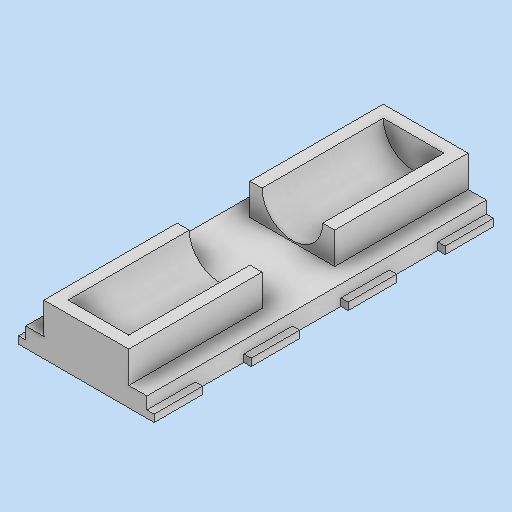
# Autodesk Inventor part: bottom plate
Saved by Autodesk Inventor 2026 (Build 300175000, 175)
## iProperties
Created: 2026-02-10
Part Number: bottom plate
Material: Generic
Document SubType Name: Modeling
Designer: mones
Density: 1 g/cm^3
Appearance: Default
Author: mones
Autodesk Inventor part; units mm, degrees
ref_plane "YZ Plane" through (0, 0, 0) normal (1, 0, 0) x (0, 1, 0)
ref_plane "XZ Plane" through (0, 0, 0) normal (0, 1, 0) x (-1, 0, 0)
ref_plane "XY Plane" through (0, 0, 0) normal (0, 0, 1) x (1, 0, 0)
sketch "Sketch1" plane through (0, 0, 0) normal (0, 1, 0) x (-1, 0, 0)
  line L0 (28, -70) -> (-28, -70)
  line L1 (-28, 70) -> (28, 70)
  line L2 (28, -70) -> (-28, 70) construction
  line L3 (-28, -70) -> (28, 70) construction
  line L4 (28, -70) -> (25, -70)
  line L5 (28, -70) -> (28, -50)
  line L6 (28, -30) -> (28, -10)
  line L7 (28, 10) -> (28, 30)
  line L8 (28, 50) -> (28, 70)
  line L9 (28, 50) -> (25, 50)
  line L10 (28, 30) -> (25, 30)
  line L11 (28, 10) -> (25, 10)
  line L12 (28, -10) -> (25, -10)
  line L13 (28, -30) -> (25, -30)
  line L14 (28, -50) -> (25, -50)
  line L15 (-28, -70) -> (-25, -70)
  line L16 (-28, 70) -> (-28, 50)
  line L17 (-28, 30) -> (-28, 10)
  line L18 (-28, -10) -> (-28, -30)
  line L19 (-28, -50) -> (-25, -50)
  line L20 (-28, -30) -> (-25, -30)
  line L21 (-28, -10) -> (-25, -10)
  line L22 (-28, 10) -> (-25, 10)
  line L23 (-28, 30) -> (-25, 30)
  line L24 (-28, 50) -> (-25, 50)
  line L25 (-28, -70) -> (-28, -50)
  line L26 (-28, -30) -> (-28, -10)
  line L27 (-28, 10) -> (-28, 30)
  line L28 (-28, 50) -> (-28, 70)
  line L29 (28, -50) -> (28, -70)
  line L30 (28, -10) -> (28, -30)
  line L31 (28, 70) -> (28, 50)
  line L32 (28, 30) -> (28, 10)
  line L33 (25, -50) -> (25, -30)
  line L34 (25, -10) -> (25, 10)
  line L35 (25, 30) -> (25, 50)
  line L36 (-25, 30) -> (-25, 50)
  line L37 (-25, -50) -> (-25, -30)
  line L38 (-25, -10) -> (-25, 10)
  point P0 (0, 0)
  dimension "d0" = 56
  dimension "d1" = 140
  dimension "d2" = 3
  constraints: 78 end point, 34 perpendicular, 25 equal length, 2 midpoint, 2 point on line, 1 horizontal
  measures "d0" distance of L0.start L0.end
  measures "d1" distance of L0.end L1.start
  measures "d2" distance of L0.start L4.end
extrude "Extrusion1" add sketch "Sketch1" along normal blind 3
sketch "Sketch2" plane through (0, 3, 0) normal (0, 1, 0) x (1, 0, 0)
  line L0 (28, -70) -> (28, -50) projected
  line L1 (28, -50) -> (25, -50) projected
  line L2 (25, -50) -> (25, -30) projected
  line L3 (25, -30) -> (28, -30) projected
  line L4 (28, -30) -> (28, -10) projected
  line L5 (28, -10) -> (25, -10) projected
  line L6 (25, -10) -> (25, 10) projected
  line L7 (25, 10) -> (28, 10) projected
  line L8 (28, 10) -> (28, 30) projected
  line L9 (28, 30) -> (25, 30) projected
  line L10 (25, 30) -> (25, 50) projected
  line L11 (25, 50) -> (28, 50) projected
  line L12 (28, 50) -> (28, 70) projected
  line L13 (28, 70) -> (-28, 70) projected
  line L14 (-28, 70) -> (-28, 50) projected
  line L15 (-28, 50) -> (-25, 50) projected
  line L16 (-25, 50) -> (-25, 30) projected
  line L17 (-25, 30) -> (-28, 30) projected
  line L18 (-28, 30) -> (-28, 10) projected
  line L19 (-28, 10) -> (-25, 10) projected
  line L20 (-25, 10) -> (-25, -10) projected
  line L21 (-25, -10) -> (-28, -10) projected
  line L22 (-28, -10) -> (-28, -30) projected
  line L23 (-28, -30) -> (-25, -30) projected
  line L24 (-25, -30) -> (-25, -50) projected
  line L25 (-25, -50) -> (-28, -50) projected
  line L26 (-28, -50) -> (-28, -70) projected
  line L27 (-28, -70) -> (28, -70) projected
  line L28 (-25, 50) -> (-25, 70)
  line L29 (-25, 70) -> (25, 70)
  line L30 (25, 70) -> (25, -70)
  line L31 (25, -70) -> (-25, -70)
  line L32 (-25, -70) -> (-25, 50)
  dimension "d19" = 50
  dimension "d20" = 50
  constraints: 10 end point, 4 point on line, 2 perpendicular
  measures "d19" distance of L28.end L29.end
  measures "d20" distance of L30.end L31.end
extrude "Extrusion2" add sketch "Sketch2" along normal blind 5 contours L27 L32 L24 L20 L16 L28 L13 L30 L10 L6 L2
sketch "Sketch3" plane through (0, 8, 0) normal (0, 1, 0) x (1, 0, 0)
  line L0 (-25, 70) -> (-25, -70) projected
  line L1 (-25, -70) -> (25, -70) projected
  line L2 (25, -70) -> (25, 70) projected
  line L3 (25, 70) -> (-25, 70) projected
  line L4 (-17.5, -70) -> (17.5, -70)
  line L5 (0, -70) -> (0, -15)
  line L6 (-17.5, 70) -> (17.5, 70)
  line L7 (0, 70) -> (0, 15)
  line L8 (-17.5, 15) -> (-17.5, 70)
  line L9 (-17.5, 70) -> (17.5, 70)
  line L10 (17.5, 70) -> (17.5, 15)
  line L11 (17.5, 15) -> (-17.5, 15)
  line L12 (-17.5, 15) -> (17.5, 70) construction
  line L13 (-17.5, 70) -> (17.5, 15) construction
  line L14 (-17.5, -70) -> (-17.5, -15)
  line L15 (-17.5, -15) -> (17.5, -15)
  line L16 (17.5, -15) -> (17.5, -70)
  line L17 (17.5, -70) -> (-17.5, -70)
  line L18 (-17.5, -70) -> (17.5, -15) construction
  line L19 (-17.5, -15) -> (17.5, -70) construction
  point P0 (0, 42.5)
  point P1 (0, -42.5)
  dimension "d23" = 35
  dimension "d24" = 55
  dimension "d25" = 35
  dimension "d26" = 55
  constraints: 32 end point, 10 midpoint, 5 parallel, 3 vertical, 2 perpendicular, 2 point on line
  measures "d23" distance of L4.start L4.end
  measures "d24" distance of L5.start L5.end
  measures "d25" distance of L6.start L6.end
  measures "d26" distance of L7.start L7.end
extrude "Extrusion3" add sketch "Sketch3" along normal blind 13 contours L3 L7 L11 L8 | L14 L15 L5 L1 | L3 L10 L11 L7 | L5 L15 L16 L1
sketch "Sketch4" plane through (17.5, 8, 15) normal (0, 0, -1) x (-1, 0, 0)
  line L0 (0, 13) -> (35, 13) projected
  arc A0 (5, 13) -> (30, 13) centre (17.5, 13) ccw
  dimension "d29" = 12.5
  constraints: 2 point on circle, 2 point on line, 1 centre point, 1 midpoint
  measures "d29" radius of A0
extrude "Extrusion4" cut sketch "Sketch4" against normal blind 50
sketch "Sketch5" plane through (-17.5, 8, -15) normal (0, 0, 1) x (1, 0, 0)
  line L0 (0, 13) -> (35, 13) projected
  arc A0 (5, 13) -> (30, 13) centre (17.5, 13) ccw
  dimension "d32" = 12.5
  constraints: 2 point on circle, 2 point on line, 1 centre point, 1 midpoint
  measures "d32" radius of A0
extrude "Extrusion5" cut sketch "Sketch5" against normal blind 50
body "Solid1"
